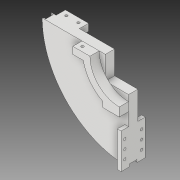
# Autodesk Inventor part: 2125B_Bearing Clamps Gear_V1
Saved by Autodesk Inventor 2020 (Build 240168000, 168)
## iProperties
Created: 2017-06-21
Part Number: 2125B_Bearing Clamps Gear_V1
Material: ABS Plastic
Document SubType Name: Modeling
Designer: MPI
Density: 1.06 g/cm^3
Appearance: Smooth - White
Mass: 4002.07 g
Surface Area: 3908.8 cm^2
Volume: 3775.53 cm^3
Author: MPI
Autodesk Inventor part; units mm, degrees
(part 1 of 3)
ref_plane "YZ Plane" through (0, 0, 0) normal (1, 0, 0) x (0, 1, 0)
ref_plane "XZ Plane" through (0, 0, 0) normal (0, 1, 0) x (-1, 0, 0)
ref_plane "XY Plane" through (0, 0, 0) normal (0, 0, 1) x (1, 0, 0)
sketch "Sketch1" plane through (0, 0, 0) normal (0, 0, 1) x (1, 0, 0)
  circle A0 centre (0, 0) radius 80.137
  line L0 (-127, -19.05) -> (-127, 19.05)
  line L1 (127, 19.05) -> (127, -19.05)
  line L2 (127, -19.05) -> (-127, 19.05) construction
  line L3 (-127, -19.05) -> (127, 19.05) construction
  line L4 (-127, 0) -> (88.9567, 0) construction
  line L5 (-127, 19.05) -> (-99.7981, 19.05)
  line L6 (99.7981, 19.05) -> (127, 19.05)
  arc A1 (-98.1276, -19.05) -> (98.1276, -19.05) centre (0, 0) ccw
  arc A2 (99.7981, 19.05) -> (-99.7981, 19.05) centre (0, 0) ccw
  line L7 (127, -19.05) -> (98.1276, -19.05)
  line L8 (-98.1276, -19.05) -> (-127, -19.05)
  dimension "d0" = 160.274
  dimension "d2" = 254
  dimension "d3" = 38.1
  dimension "d137" = 101.6
  dimension "d138" = 127
  dimension "d139" = 19.05
  dimension "d155" = 21.463
  constraints: 18 end point, 7 parallel, 4 point on circle, 3 centre point, 3 midpoint, 2 coincident, 2 horizontal, 2 perpendicular
  measures "d0" diameter of A0
  measures "d2" distance of L1.end L0.start
  measures "d3" distance of L0.start L0.end
  measures "d137" radius of A2
  measures "d138" distance from line of A0.centre L0
  measures "d139" distance from line of A0.centre L5
  measures "d155" radial gap between concentric circles of A2 A0
extrude "Extrusion1" add sketch "Sketch1" along normal blind 25.4
sketch "Sketch2" plane through (99.7981, 19.05, 0) normal (0, 1, 0) x (1, 0, 0)
  line L0 (27.2019, 0) -> (0, 0) projected
  line L1 (0, 0) -> (0, -25.4) projected
  line L2 (27.2019, -25.4) -> (0, -25.4) projected
  line L3 (27.2019, 0) -> (27.2019, -25.4) projected
  line L4 (27.2019, -12.7) -> (0, -12.7) construction
  line L5 (13.601, -25.4) -> (13.601, 0) construction
  circle A0 centre (13.601, -12.7) radius 3.3782
  point P0 (-99.7981, 0)
  dimension "d6" = 6.7564
  constraints: 5 midpoint, 4 end point, 1 centre point
  measures "d6" diameter of A0
extrude "Extrusion2" cut sketch "Sketch2" against normal blind 38.1 contours A0
mirror "Mirror1" about plane through (0, 0, 0) normal (1, 0, 0) of "Extrusion2"
sketch "Sketch4" plane through (0, 0, 0) normal (0, 0, -1) x (-1, 0, 0)
  arc A0 (99.7981, 19.05) -> (-99.7981, 19.05) centre (0, 0) ccw projected
  line L0 (-63.5, -63.5) -> (63.5, -63.5)
  line L1 (63.5, -63.5) -> (63.5, 63.5)
  line L2 (63.5, 63.5) -> (-63.5, 63.5)
  line L3 (-63.5, 63.5) -> (-63.5, -63.5)
  line L4 (-63.5, -63.5) -> (63.5, 63.5) construction
  line L5 (-89.8026, 89.8026) -> (89.8026, -89.8026) construction
  circle A1 centre (0, 0) radius 228.9048
  circle A2 centre (0, 0) radius 146.8598 construction
  line L6 (-9.525, 228.7065) -> (-6.111, 146.7326) construction
  line L7 (0, 146.8598) -> (0, 125.8958) construction
  arc A3 (0, 125.8958) -> (-4.7163, 125.8085) centre (-0.0298, 0.0716) ccw construction
  line L8 (-2.3813, 228.8924) -> (-2.3813, 146.8405)
  line L9 (-6.7286, 228.824) -> (-6.7278, 228.8059)
  arc A4 (-5.196, 124.7614) -> (-9.4765, 124.5104) centre (-0.0298, 0.0716) ccw
  arc A5 (-2.3813, 146.8405) -> (-4.0495, 146.8039) centre (0, 0) ccw
  line L10 (-7.1437, 228.7933) -> (-5.8965, 146.7413)
  dimension "d11" = 127
  dimension "d12" = 127
  dimension "d28" = 457.8096
  dimension "d30" = 82.045
  dimension "d33" = 9.525
  dimension "d34" = 20.964
  dimension "d35" = 81.974
  dimension "d36" = 2.3813
  dimension "d39" = 2.3813
  dimension "d40" = 82.052
  dimension "d41" = 82.052
  constraints: 22 end point, 15 point on circle, 5 centre point, 3 parallel, 2 coincident, 2 concentric, 2 line through centre, 2 midpoint, 1 horizontal, 1 perpendicular, 1 point on line, 1 vertical
  measures "d11" distance of L2.end L1.end
  measures "d12" distance of L1.end L0.end
  measures "d28" diameter of A1
  measures "d30" radial gap between concentric circles of A1 A2
  measures "d33" horizontal distance of L7.end L6.start
  measures "d34" distance of L7.start L7.end
  measures "d35" vertical distance of L6.start L6.end
  measures "d36" distance between parallel lines of L8 L7
  measures "d39" horizontal distance of L6.start L10.start
  measures "d40" distance of L8.start L8.end
  measures "d41" vertical distance of L10.start L10.end
extrude "Extrusion4" add sketch "Sketch4" along normal blind 25.4 separate body
sketch "Sketch8" plane through (0, 0, 0) normal (0, 0, 1) x (1, 0, 0)
  circle A0 centre (0, 0) radius 228.9048 projected
  arc A1 (9.5229, 228.7066) -> (0, 228.9048) centre (0, 0) ccw
  line L0 (4.7625, 228.8553) -> (4.7182, 226.7257) construction
  circle A2 centre (0, 0) radius 226.7801 construction
  line L1 (-6.0145, 226.7003) -> (3.1685, 226.758) construction
  line L2 (9.5229, 228.7066) -> (9.4345, 226.5838) construction
  line L3 (9.4345, 226.5838) -> (6.2678, 226.6935) construction
  line L4 (6.2678, 226.6935) -> (7.1073, 228.7944)
  line L5 (3.1685, 226.758) -> (2.4172, 228.892)
  arc A3 (99.7981, 19.05) -> (-99.7981, 19.05) centre (0, 0) ccw projected
  line L6 (7.1073, 228.7944) -> (0, 0) construction
  line L7 (0, 0) -> (2.4172, 228.892) construction
  line L8 (6.2678, 226.6935) -> (3.1685, 226.758)
  point P0 (12.7, 94.3995)
  point P1 (-12.7, 94.3995)
  dimension "d42" = 9.525
  dimension "d43" = 2.13
  dimension "d46" = 3.1686
  dimension "d52" = 20
  dimension "d53" = 20
  dimension "d55" = 3.1
  constraints: 18 end point, 13 point on circle, 2 centre point, 2 line through centre, 1 concentric, 1 midpoint, 1 vertical alignment, 1 other
  measures "d42" distance of A0.end L2.start
  measures "d43" distance of L0.end L0.start
  measures "d46" distance of L2.end L3.end
  measures "d52" angle of L5 L7
  measures "d53" angle of L6 L4
  measures "d55" distance of L1.end L3.end
extrude "Extrusion6" cut sketch "Sketch8" against normal blind 25.4 contours L4 L8 L5 A0 picked at (4.4724, 227.4406) bodies 2
pattern_circular "Circular Pattern1" count 152 over 360 about axis through (0, 0, 0) along (0, 0, -1) of "Extrusion6" bodies 2
sketch "Sketch9" plane through (0, 0, 25.4) normal (0, 0, 1) x (1, 0, 0)
  circle A0 centre (-78.9498, 78.9498) radius 4.7625 projected
  circle A1 centre (78.9498, 78.9498) radius 4.7625 projected
  line L0 (127, -19.05) -> (127, 19.05) projected
  line L1 (127, 19.05) -> (99.7981, 19.05) projected
  line L2 (94.3995, 12.7) -> (94.3995, 94.3995) projected
  line L3 (94.3995, 94.3995) -> (12.7, 94.3995) projected
  arc A2 (99.7981, 19.05) -> (-99.7981, 19.05) centre (0, 0) ccw projected
  line L4 (-12.7, 94.3995) -> (-94.3995, 94.3995) projected
  line L5 (-94.3995, 94.3995) -> (-94.3995, 12.7) projected
  line L6 (-99.7981, 19.05) -> (-127, 19.05) projected
  line L7 (-127, 19.05) -> (-127, -19.05) projected
  line L8 (-127, 0) -> (127, 0)
  constraints: 2 end point, 2 midpoint, 3 other
extrude "Extrusion7" cut sketch "Sketch9" against normal blind 25.4 contours L8 L7 L6 A2 L1 L0 bodies 1
sketch "Sketch11" plane through (0, 0, 0) normal (0, 0, 1) x (1, 0, 0)
  line L0 (-63.5, 63.5) -> (63.5, 63.5) projected
  line L1 (0, 63.5) -> (0, 139.7) construction
  line L2 (0, 63.5) -> (76.2, 63.5) construction
  line L3 (0, 139.7) -> (25.4, 139.7) construction
  line L4 (-25.4, 127) -> (25.4, 127) construction
  line L5 (25.4, 127) -> (25.4, 152.4)
  line L6 (25.4, 152.4) -> (-25.4, 152.4) construction
  line L7 (-25.4, 152.4) -> (-25.4, 127)
  line L8 (-25.4, 127) -> (25.4, 152.4) construction
  line L9 (25.4, 127) -> (-25.4, 152.4) construction
  line L10 (0, 139.7) -> (0, 133.35)
  line L11 (0, 133.35) -> (25.4, 127)
  line L12 (0, 133.35) -> (-25.4, 127)
  line L13 (0, 146.05) -> (25.4, 152.4)
  line L14 (0, 146.05) -> (-25.4, 152.4)
  line L15 (-25.4, 127) -> (-25.4, 107.95) construction
  line L16 (-25.4, 107.95) -> (25.4, 107.95) construction
  circle A0 centre (-25.4, 107.95) radius 4.4323
  circle A1 centre (25.4, 107.95) radius 4.4323
  line L17 (-25.4, 139.7) -> (25.4, 139.7) construction
  circle A2 centre (-25.4, 171.45) radius 4.4323
  circle A3 centre (25.4, 171.45) radius 4.4323
  dimension "d65" = 76.2
  dimension "d66" = 90
  dimension "d67" = 25.4
  dimension "d68" = 25.4
  dimension "d69" = 6.35
  dimension "d127" = 19.05
  dimension "d128" = 50.8
  dimension "d129" = 90
  dimension "d130" = 8.8646
  dimension "d131" = 8.8646
  dimension "d132" = 25.4
  constraints: 34 end point, 4 centre point, 4 midpoint, 4 perpendicular, 3 parallel, 3 symmetric about line, 2 coincident, 2 vertical, 1 collinear, 1 horizontal, 1 point on line, 2 other
  measures "d65" distance of L1.start L1.end
  measures "d66" angle of L2 L1
  measures "d67" distance of L1.end L3.end
  measures "d68" distance of L5.end L4.end
  measures "d69" distance of L1.end L10.end
  measures "d127" distance of L4.start L15.end
  measures "d128" distance of L15.end L16.end
  measures "d129" angle of L16 L15
  measures "d130" diameter of A0
  measures "d131" diameter of A1
  measures "d132" distance from line of L16.end L1
extrude "Extrusion9" cut sketch "Sketch11" against normal blind 21.59 contours L11 L12 L7 L14 L13 L5 | A2 | A3 bodies 2
sketch "Sketch17" plane through (0, 0, 0) normal (0, 0, 1) x (1, 0, 0)
  line L0 (-15.5678, 226.2451) -> (-16.4928, 228.3099) projected
  arc A0 (-16.4928, 228.3099) -> (-21.2475, 227.9165) centre (0, 0) ccw projected
  line L1 (-21.2475, 227.9165) -> (-21.8206, 225.7279) projected
  line L2 (-21.8206, 225.7279) -> (-24.9041, 225.4085) projected
  line L3 (-24.9041, 225.4085) -> (-25.9136, 227.4333) projected
  arc A1 (-25.9136, 227.4333) -> (-30.648, 226.8438) centre (0, 0) ccw projected
  line L4 (-30.648, 226.8438) -> (-31.1302, 224.6333) projected
  line L5 (-31.1302, 224.6333) -> (-34.1978, 224.1868) projected
  line L6 (-34.1978, 224.1868) -> (-35.2902, 226.1681) projected
  arc A2 (-35.2902, 226.1681) -> (-39.9961, 225.3835) centre (0, 0) ccw projected
  line L7 (-39.9961, 225.3835) -> (-40.3865, 223.155) projected
  line L8 (-40.3865, 223.155) -> (-43.4331, 222.5821) projected
  line L9 (-43.4331, 222.5821) -> (-44.6064, 224.5165) projected
  arc A3 (-44.6064, 224.5165) -> (-49.2759, 223.5381) centre (0, 0) ccw projected
  line L10 (-49.2759, 223.5381) -> (-49.5739, 221.2954) projected
  line L11 (-49.5739, 221.2954) -> (-52.5942, 220.5971) projected
  line L12 (-52.5942, 220.5971) -> (-53.8464, 222.4814) projected
  arc A4 (-53.8464, 222.4814) -> (-58.4715, 221.3108) centre (0, 0) ccw projected
  line L13 (-58.4715, 221.3108) -> (-58.6766, 219.0577) projected
  line L14 (-58.6766, 219.0577) -> (-61.6655, 218.2352) projected
  line L15 (-61.6655, 218.2352) -> (-62.9945, 220.0661) projected
  arc A5 (-62.9945, 220.0661) -> (-67.5672, 218.7055) centre (0, 0) ccw projected
  line L16 (-67.5672, 218.7055) -> (-67.679, 216.4458) projected
  line L17 (-67.679, 216.4458) -> (-70.6313, 215.5004) projected
  line L18 (-70.6313, 215.5004) -> (-72.0349, 217.2749) projected
  arc A6 (-72.0349, 217.2749) -> (-76.5475, 215.7264) centre (0, 0) ccw projected
  line L19 (-76.5475, 215.7264) -> (-76.5658, 213.464) projected
  line L20 (-76.5658, 213.464) -> (-79.4766, 212.3975) projected
  line L21 (-79.4766, 212.3975) -> (-80.9522, 214.1125) projected
  arc A7 (-80.9522, 214.1125) -> (-85.397, 212.3788) centre (0, 0) ccw projected
  line L22 (-85.397, 212.3788) -> (-85.3218, 210.1176) projected
  line L23 (-85.3218, 210.1176) -> (-88.186, 208.9317) projected
  line L24 (-88.186, 208.9317) -> (-89.7313, 210.5842) projected
  arc A8 (-89.7313, 210.5842) -> (-94.1006, 208.6684) centre (0, 0) ccw projected
  line L25 (-94.1006, 208.6684) -> (-93.932, 206.4122) projected
  line L26 (-93.932, 206.4122) -> (-96.7448, 205.1089) projected
  line L27 (-96.7448, 205.1089) -> (-98.357, 206.6962) projected
  arc A9 (-98.357, 206.6962) -> (-102.6434, 204.6014) centre (0, 0) ccw projected
  line L28 (-102.6434, 204.6014) -> (-102.3818, 202.3541) projected
  line L29 (-102.3818, 202.3541) -> (-105.1382, 200.9357) projected
  line L30 (-105.1382, 200.9357) -> (-106.8147, 202.455) projected
  arc A10 (-106.8147, 202.455) -> (-111.0109, 200.1849) centre (0, 0) ccw projected
  line L31 (-111.0109, 200.1849) -> (-110.6566, 197.9503) projected
  line L32 (-110.6566, 197.9503) -> (-113.3521, 196.4192) projected
  line L33 (-113.3521, 196.4192) -> (-115.0899, 197.8679) projected
  arc A11 (-115.0899, 197.8679) -> (-119.1887, 195.4264) centre (0, 0) ccw projected
  line L34 (-119.1887, 195.4264) -> (-118.7423, 193.2084) projected
  line L35 (-118.7423, 193.2084) -> (-121.3723, 191.5672) projected
  line L36 (-121.3723, 191.5672) -> (-123.1685, 192.9428) projected
  arc A12 (-123.1685, 192.9428) -> (-127.1629, 190.3339) centre (0, 0) ccw projected
  line L37 (-127.1629, 190.3339) -> (-126.6252, 188.1363) projected
  line L38 (-126.6252, 188.1363) -> (-129.1851, 186.3878) projected
  line L39 (-129.1851, 186.3878) -> (-131.0366, 187.6881) projected
  arc A13 (-131.0366, 187.6881) -> (-134.9198, 184.9163) centre (0, 0) ccw projected
  line L40 (-134.9198, 184.9163) -> (-134.2918, 182.7428) projected
  line L41 (-134.2918, 182.7428) -> (-136.7772, 180.89) projected
  line L42 (-136.7772, 180.89) -> (-138.6809, 182.1127) projected
  arc A14 (-138.6809, 182.1127) -> (-142.4462, 179.1828) centre (0, 0) ccw projected
  line L43 (-142.4462, 179.1828) -> (-141.7289, 177.0371) projected
  line L44 (-141.7289, 177.0371) -> (-144.1357, 175.0832) projected
  line L45 (-144.1357, 175.0832) -> (-146.0882, 176.2261) projected
  arc A15 (-146.0882, 176.2261) -> (-149.7292, 173.1432) centre (0, 0) ccw projected
  line L46 (-149.7292, 173.1432) -> (-148.9239, 171.0289) projected
  line L47 (-148.9239, 171.0289) -> (-151.2478, 168.9772) projected
  line L48 (-151.2478, 168.9772) -> (-153.246, 170.0385) projected
  arc A16 (-153.246, 170.0385) -> (-156.7565, 166.8077) centre (0, 0) ccw projected
  line L49 (-156.7565, 166.8077) -> (-155.8644, 164.7285) projected
  line L50 (-155.8644, 164.7285) -> (-158.1016, 162.5826) projected
  line L51 (-158.1016, 162.5826) -> (-160.1419, 163.5603) projected
  arc A17 (-160.1419, 163.5603) -> (-163.5159, 160.1873) centre (0, 0) ccw projected
  line L52 (-163.5159, 160.1873) -> (-162.5387, 158.1467) projected
  line L53 (-162.5387, 158.1467) -> (-164.6853, 155.9101) projected
  line L54 (-164.6853, 155.9101) -> (-166.7642, 156.8028) projected
  arc A18 (-166.7642, 156.8028) -> (-169.9959, 153.2931) centre (0, 0) ccw projected
  line L55 (-169.9959, 153.2931) -> (-168.9353, 151.2947) projected
  line L56 (-168.9353, 151.2947) -> (-170.9876, 148.9713) projected
  line L57 (-170.9876, 148.9713) -> (-173.1016, 149.7773) projected
  arc A19 (-173.1016, 149.7773) -> (-176.1856, 146.1371) centre (0, 0) ccw projected
  line L58 (-176.1856, 146.1371) -> (-175.0432, 144.1842) projected
  line L59 (-175.0432, 144.1842) -> (-176.9977, 141.778) projected
  line L60 (-176.9977, 141.778) -> (-179.1433, 142.4959) projected
  arc A20 (-179.1433, 142.4959) -> (-182.0742, 138.7314) centre (0, 0) ccw projected
  line L61 (-182.0742, 138.7314) -> (-180.8521, 136.8274) projected
  line L62 (-180.8521, 136.8274) -> (-182.7055, 134.3425) projected
  line L63 (-182.7055, 134.3425) -> (-184.8789, 134.9711) projected
  arc A21 (-184.8789, 134.9711) -> (-187.6517, 131.0887) centre (0, 0) ccw projected
  line L64 (-187.6517, 131.0887) -> (-186.352, 129.2368) projected
  line L65 (-186.352, 129.2368) -> (-188.1011, 126.6774) projected
  line L66 (-188.1011, 126.6774) -> (-190.2987, 127.2157) projected
  arc A22 (-190.2987, 127.2157) -> (-192.9086, 123.222) centre (0, 0) ccw projected
  line L67 (-192.9086, 123.222) -> (-191.5335, 121.4254) projected
  line L68 (-191.5335, 121.4254) -> (-193.1754, 118.7959) projected
  line L69 (-193.1754, 118.7959) -> (-195.3933, 119.2429) projected
  arc A23 (-195.3933, 119.2429) -> (-197.836, 115.1448) centre (0, 0) ccw projected
  line L70 (-197.836, 115.1448) -> (-196.3878, 113.4066) projected
  line L71 (-196.3878, 113.4066) -> (-197.9196, 110.7115) projected
  line L72 (-197.9196, 110.7115) -> (-200.1541, 111.0664) projected
  arc A24 (-200.1541, 111.0664) -> (-202.4254, 106.8709) centre (0, 0) ccw projected
  line L73 (-202.4254, 106.8709) -> (-200.9065, 105.194) projected
  line L74 (-200.9065, 105.194) -> (-202.3257, 102.4379) projected
  line L75 (-202.3257, 102.4379) -> (-204.5729, 102.7002) projected
  arc A25 (-204.5729, 102.7002) -> (-206.6689, 98.4143) centre (0, 0) ccw projected
  line L76 (-206.6689, 98.4143) -> (-205.0821, 96.8017) projected
  line L77 (-205.0821, 96.8017) -> (-206.3861, 93.9893) projected
  line L78 (-206.3861, 93.9893) -> (-208.6422, 94.1585) projected
  arc A26 (-208.6422, 94.1585) -> (-210.5593, 89.7897) centre (0, 0) ccw projected
  line L79 (-210.5593, 89.7897) -> (-208.9072, 88.244) projected
  line L80 (-208.9072, 88.244) -> (-210.0939, 85.3801) projected
  line L81 (-210.0939, 85.3801) -> (-212.3551, 85.4559) projected
  arc A27 (-212.3551, 85.4559) -> (-214.09, 81.0116) centre (0, 0) ccw projected
  line L82 (-214.09, 81.0116) -> (-212.3754, 79.5355) projected
  line L83 (-212.3754, 79.5355) -> (-213.4428, 76.625) projected
  line L84 (-213.4428, 76.625) -> (-215.7052, 76.6074) projected
  arc A28 (-215.7052, 76.6074) -> (-217.2549, 72.0952) centre (0, 0) ccw projected
  line L85 (-217.2549, 72.0952) -> (-215.4808, 70.6911) projected
  line L86 (-215.4808, 70.6911) -> (-216.427, 67.7391) projected
  line L87 (-216.427, 67.7391) -> (-218.6867, 67.6279) projected
  arc A29 (-218.6867, 67.6279) -> (-220.0486, 63.0555) centre (0, 0) ccw projected
  line L88 (-220.0486, 63.0555) -> (-218.218, 61.726) projected
  line L89 (-218.218, 61.726) -> (-219.0414, 58.7374) projected
  line L90 (-219.0414, 58.7374) -> (-221.2946, 58.5329) projected
  arc A30 (-221.2946, 58.5329) -> (-222.4664, 53.9082) centre (0, 0) ccw projected
  line L91 (-222.4664, 53.9082) -> (-220.5825, 52.6554) projected
  line L92 (-220.5825, 52.6554) -> (-221.2816, 49.6353) projected
  line L93 (-221.2816, 49.6353) -> (-223.5244, 49.3379) projected
  arc A31 (-223.5244, 49.3379) -> (-224.5042, 44.6687) centre (0, 0) ccw projected
  line L94 (-224.5042, 44.6687) -> (-222.57, 43.4949) projected
  line L95 (-222.57, 43.4949) -> (-223.1438, 40.4484) projected
  line L96 (-223.1438, 40.4484) -> (-225.3724, 40.0586) projected
  arc A32 (-225.3724, 40.0586) -> (-226.1583, 35.3529) centre (0, 0) ccw projected
  line L97 (-226.1583, 35.3529) -> (-224.1773, 34.26) projected
  line L98 (-224.1773, 34.26) -> (-224.6247, 31.1925) projected
  line L99 (-224.6247, 31.1925) -> (-226.8353, 30.7109) projected
  arc A33 (-226.8353, 30.7109) -> (-227.4261, 25.9767) centre (0, 0) ccw projected
  line L100 (-227.4261, 25.9767) -> (-225.4016, 24.9666) projected
  line L101 (-225.4016, 24.9666) -> (-225.7218, 21.8832) projected
  line L102 (-225.7218, 21.8832) -> (-227.9106, 21.3107) projected
  arc A34 (-227.9106, 21.3107) -> (-228.3053, 16.5561) centre (0, 0) ccw projected
  line L103 (-228.3053, 16.5561) -> (-226.2408, 15.6306) projected
  line L104 (-226.2408, 15.6306) -> (-226.4333, 12.5366) projected
  line L105 (-226.4333, 12.5366) -> (-228.5966, 11.8741) projected
  arc A35 (-228.5966, 11.8741) -> (-228.7944, 7.1073) centre (0, 0) ccw projected
  line L106 (-228.7944, 7.1073) -> (-226.6935, 6.2678) projected
  line L107 (-226.6935, 6.2678) -> (-226.758, 3.1685) projected
  line L108 (-226.758, 3.1685) -> (-228.892, 2.4172) projected
  arc A36 (-228.892, 2.4172) -> (-228.8927, -2.3537) centre (0, 0) ccw projected
  line L109 (-228.8927, -2.3537) -> (-226.7588, -3.1056) projected
  line L110 (-226.7588, -3.1056) -> (-226.6952, -6.205) projected
  line L111 (-226.6952, -6.205) -> (-228.7964, -7.0438) projected
  arc A37 (-228.7964, -7.0438) -> (-228.5999, -11.8107) centre (0, 0) ccw projected
  line L112 (-228.5999, -11.8107) -> (-226.4368, -12.4738) projected
  line L113 (-226.4368, -12.4738) -> (-226.2451, -15.5678) projected
  line L114 (-226.2451, -15.5678) -> (-228.3099, -16.4928) projected
  arc A38 (-228.3099, -16.4928) -> (-227.9165, -21.2475) centre (0, 0) ccw projected
  line L115 (-227.9165, -21.2475) -> (-225.7279, -21.8206) projected
  line L116 (-225.7279, -21.8206) -> (-225.4085, -24.9041) projected
  line L117 (-225.4085, -24.9041) -> (-227.4333, -25.9136) projected
  arc A39 (-227.4333, -25.9136) -> (-226.8438, -30.648) centre (0, 0) ccw projected
  line L118 (-226.8438, -30.648) -> (-224.6333, -31.1302) projected
  line L119 (-224.6333, -31.1302) -> (-224.1868, -34.1978) projected
  line L120 (-224.1868, -34.1978) -> (-226.1681, -35.2902) projected
  arc A40 (-226.1681, -35.2902) -> (-225.3835, -39.9961) centre (0, 0) ccw projected
  line L121 (-225.3835, -39.9961) -> (-223.155, -40.3865) projected
  line L122 (-223.155, -40.3865) -> (-222.5821, -43.4331) projected
  line L123 (-222.5821, -43.4331) -> (-224.5165, -44.6064) projected
  arc A41 (-224.5165, -44.6064) -> (-223.5381, -49.2759) centre (0, 0) ccw projected
  line L124 (-223.5381, -49.2759) -> (-221.2954, -49.5739) projected
  line L125 (-221.2954, -49.5739) -> (-220.5971, -52.5942) projected
  line L126 (-220.5971, -52.5942) -> (-222.4814, -53.8464) projected
  arc A42 (-222.4814, -53.8464) -> (-221.3108, -58.4715) centre (0, 0) ccw projected
  line L127 (-221.3108, -58.4715) -> (-219.0577, -58.6766) projected
  line L128 (-219.0577, -58.6766) -> (-218.2352, -61.6655) projected
  line L129 (-218.2352, -61.6655) -> (-220.0661, -62.9945) projected
  arc A43 (-220.0661, -62.9945) -> (-218.7055, -67.5672) centre (0, 0) ccw projected
  line L130 (-218.7055, -67.5672) -> (-216.4458, -67.679) projected
  line L131 (-216.4458, -67.679) -> (-215.5004, -70.6313) projected
  line L132 (-215.5004, -70.6313) -> (-217.2749, -72.0349) projected
  arc A44 (-217.2749, -72.0349) -> (-215.7264, -76.5475) centre (0, 0) ccw projected
  line L133 (-215.7264, -76.5475) -> (-213.464, -76.5658) projected
  line L134 (-213.464, -76.5658) -> (-212.3975, -79.4766) projected
  line L135 (-212.3975, -79.4766) -> (-214.1125, -80.9522) projected
  arc A45 (-214.1125, -80.9522) -> (-212.3788, -85.397) centre (0, 0) ccw projected
  line L136 (-212.3788, -85.397) -> (-210.1176, -85.3218) projected
  line L137 (-210.1176, -85.3218) -> (-208.9317, -88.186) projected
  line L138 (-208.9317, -88.186) -> (-210.5842, -89.7313) projected
  arc A46 (-210.5842, -89.7313) -> (-208.6684, -94.1006) centre (0, 0) ccw projected
  line L139 (-208.6684, -94.1006) -> (-206.4122, -93.932) projected
  line L140 (-206.4122, -93.932) -> (-205.1089, -96.7448) projected
  line L141 (-205.1089, -96.7448) -> (-206.6962, -98.357) projected
  arc A47 (-206.6962, -98.357) -> (-204.6014, -102.6434) centre (0, 0) ccw projected
  line L142 (-204.6014, -102.6434) -> (-202.3541, -102.3818) projected
  line L143 (-202.3541, -102.3818) -> (-200.9357, -105.1382) projected
  line L144 (-200.9357, -105.1382) -> (-202.455, -106.8147) projected
  arc A48 (-202.455, -106.8147) -> (-200.1849, -111.0109) centre (0, 0) ccw projected
  line L145 (-200.1849, -111.0109) -> (-197.9503, -110.6566) projected
  line L146 (-197.9503, -110.6566) -> (-196.4192, -113.3521) projected
  line L147 (-196.4192, -113.3521) -> (-197.8679, -115.0899) projected
  arc A49 (-197.8679, -115.0899) -> (-195.4264, -119.1887) centre (0, 0) ccw projected
  line L148 (-195.4264, -119.1887) -> (-193.2084, -118.7423) projected
  line L149 (-193.2084, -118.7423) -> (-191.5672, -121.3723) projected
  line L150 (-191.5672, -121.3723) -> (-192.9428, -123.1685) projected
  arc A50 (-192.9428, -123.1685) -> (-190.3339, -127.1629) centre (0, 0) ccw projected
  line L151 (-190.3339, -127.1629) -> (-188.1363, -126.6252) projected
  line L152 (-188.1363, -126.6252) -> (-186.3878, -129.1851) projected
  line L153 (-186.3878, -129.1851) -> (-187.6881, -131.0366) projected
  arc A51 (-187.6881, -131.0366) -> (-184.9163, -134.9198) centre (0, 0) ccw projected
  line L154 (-184.9163, -134.9198) -> (-182.7428, -134.2918) projected
  line L155 (-182.7428, -134.2918) -> (-180.89, -136.7772) projected
  line L156 (-180.89, -136.7772) -> (-182.1127, -138.6809) projected
  arc A52 (-182.1127, -138.6809) -> (-179.1828, -142.4462) centre (0, 0) ccw projected
  line L157 (-179.1828, -142.4462) -> (-177.0371, -141.7289) projected
  line L158 (-177.0371, -141.7289) -> (-175.0832, -144.1357) projected
  line L159 (-175.0832, -144.1357) -> (-176.2261, -146.0882) projected
  arc A53 (-176.2261, -146.0882) -> (-173.1432, -149.7292) centre (0, 0) ccw projected
  line L160 (-173.1432, -149.7292) -> (-171.0289, -148.9239) projected
  line L161 (-171.0289, -148.9239) -> (-168.9772, -151.2478) projected
  line L162 (-168.9772, -151.2478) -> (-170.0385, -153.246) projected
  arc A54 (-170.0385, -153.246) -> (-166.8077, -156.7565) centre (0, 0) ccw projected
  line L163 (-166.8077, -156.7565) -> (-164.7285, -155.8644) projected
  line L164 (-164.7285, -155.8644) -> (-162.5826, -158.1016) projected
  line L165 (-162.5826, -158.1016) -> (-163.5603, -160.1419) projected
  arc A55 (-163.5603, -160.1419) -> (-160.1873, -163.5159) centre (0, 0) ccw projected
  line L166 (-160.1873, -163.5159) -> (-158.1467, -162.5387) projected
  line L167 (-158.1467, -162.5387) -> (-155.9101, -164.6853) projected
  line L168 (-155.9101, -164.6853) -> (-156.8028, -166.7642) projected
  arc A56 (-156.8028, -166.7642) -> (-153.2931, -169.9959) centre (0, 0) ccw projected
  line L169 (-153.2931, -169.9959) -> (-151.2947, -168.9353) projected
  line L170 (-151.2947, -168.9353) -> (-148.9713, -170.9876) projected
  line L171 (-148.9713, -170.9876) -> (-149.7773, -173.1016) projected
  arc A57 (-149.7773, -173.1016) -> (-146.1371, -176.1856) centre (0, 0) ccw projected
  line L172 (-146.1371, -176.1856) -> (-144.1842, -175.0432) projected
  line L173 (-144.1842, -175.0432) -> (-141.778, -176.9977) projected
  line L174 (-141.778, -176.9977) -> (-142.4959, -179.1433) projected
  arc A58 (-142.4959, -179.1433) -> (-138.7314, -182.0742) centre (0, 0) ccw projected
  line L175 (-138.7314, -182.0742) -> (-136.8274, -180.8521) projected
  line L176 (-136.8274, -180.8521) -> (-134.3425, -182.7055) projected
  line L177 (-134.3425, -182.7055) -> (-134.9711, -184.8789) projected
  arc A59 (-134.9711, -184.8789) -> (-131.0887, -187.6517) centre (0, 0) ccw projected
  line L178 (-131.0887, -187.6517) -> (-129.2368, -186.352) projected
  line L179 (-129.2368, -186.352) -> (-126.6774, -188.1011) projected
  line L180 (-126.6774, -188.1011) -> (-127.2157, -190.2987) projected
  arc A60 (-127.2157, -190.2987) -> (-123.222, -192.9086) centre (0, 0) ccw projected
  line L181 (-123.222, -192.9086) -> (-121.4254, -191.5335) projected
  line L182 (-121.4254, -191.5335) -> (-118.7959, -193.1754) projected
  line L183 (-118.7959, -193.1754) -> (-119.2429, -195.3933) projected
  arc A61 (-119.2429, -195.3933) -> (-115.1448, -197.836) centre (0, 0) ccw projected
  line L184 (-115.1448, -197.836) -> (-113.4066, -196.3878) projected
  line L185 (-113.4066, -196.3878) -> (-110.7115, -197.9196) projected
  line L186 (-110.7115, -197.9196) -> (-111.0664, -200.1541) projected
  arc A62 (-111.0664, -200.1541) -> (-106.8709, -202.4254) centre (0, 0) ccw projected
  line L187 (-106.8709, -202.4254) -> (-105.194, -200.9065) projected
  line L188 (-105.194, -200.9065) -> (-102.4379, -202.3257) projected
  line L189 (-102.4379, -202.3257) -> (-102.7002, -204.5729) projected
  arc A63 (-102.7002, -204.5729) -> (-98.4143, -206.6689) centre (0, 0) ccw projected
  line L190 (-98.4143, -206.6689) -> (-96.8017, -205.0821) projected
  line L191 (-96.8017, -205.0821) -> (-93.9893, -206.3861) projected
  line L192 (-93.9893, -206.3861) -> (-94.1585, -208.6422) projected
  arc A64 (-94.1585, -208.6422) -> (-89.7897, -210.5593) centre (0, 0) ccw projected
  line L193 (-89.7897, -210.5593) -> (-88.244, -208.9072) projected
  line L194 (-88.244, -208.9072) -> (-85.3801, -210.0939) projected
  line L195 (-85.3801, -210.0939) -> (-85.4559, -212.3551) projected
  arc A65 (-85.4559, -212.3551) -> (-81.0116, -214.09) centre (0, 0) ccw projected
  line L196 (-81.0116, -214.09) -> (-79.5355, -212.3754) projected
  line L197 (-79.5355, -212.3754) -> (-76.625, -213.4428) projected
  line L198 (-76.625, -213.4428) -> (-76.6074, -215.7052) projected
  arc A66 (-76.6074, -215.7052) -> (-72.0952, -217.2549) centre (0, 0) ccw projected
  line L199 (-72.0952, -217.2549) -> (-70.6911, -215.4808) projected
  line L200 (-70.6911, -215.4808) -> (-67.7391, -216.427) projected
  line L201 (-67.7391, -216.427) -> (-67.6279, -218.6867) projected
  arc A67 (-67.6279, -218.6867) -> (-63.0555, -220.0486) centre (0, 0) ccw projected
  line L202 (-63.0555, -220.0486) -> (-61.726, -218.218) projected
  line L203 (-61.726, -218.218) -> (-58.7374, -219.0414) projected
  line L204 (-58.7374, -219.0414) -> (-58.5329, -221.2946) projected
  arc A68 (-58.5329, -221.2946) -> (-53.9082, -222.4664) centre (0, 0) ccw projected
  line L205 (-53.9082, -222.4664) -> (-52.6554, -220.5825) projected
  line L206 (-52.6554, -220.5825) -> (-49.6353, -221.2816) projected
  line L207 (-49.6353, -221.2816) -> (-49.3379, -223.5244) projected
  arc A69 (-49.3379, -223.5244) -> (-44.6687, -224.5042) centre (0, 0) ccw projected
  line L208 (-44.6687, -224.5042) -> (-43.4949, -222.57) projected
  line L209 (-43.4949, -222.57) -> (-40.4484, -223.1438) projected
  line L210 (-40.4484, -223.1438) -> (-40.0586, -225.3724) projected
  arc A70 (-40.0586, -225.3724) -> (-35.3529, -226.1583) centre (0, 0) ccw projected
  line L211 (-35.3529, -226.1583) -> (-34.26, -224.1773) projected
  line L212 (-34.26, -224.1773) -> (-31.1925, -224.6247) projected
  line L213 (-31.1925, -224.6247) -> (-30.7109, -226.8353) projected
  arc A71 (-30.7109, -226.8353) -> (-25.9767, -227.4261) centre (0, 0) ccw projected
  line L214 (-25.9767, -227.4261) -> (-24.9666, -225.4016) projected
  line L215 (-24.9666, -225.4016) -> (-21.8832, -225.7218) projected
  line L216 (-21.8832, -225.7218) -> (-21.3107, -227.9106) projected
  arc A72 (-21.3107, -227.9106) -> (-16.5561, -228.3053) centre (0, 0) ccw projected
  line L217 (-16.5561, -228.3053) -> (-15.6306, -226.2408) projected
  line L218 (-15.6306, -226.2408) -> (-12.5366, -226.4333) projected
  line L219 (-12.5366, -226.4333) -> (-11.8741, -228.5966) projected
  arc A73 (-11.8741, -228.5966) -> (-7.1073, -228.7944) centre (0, 0) ccw projected
  line L220 (-7.1073, -228.7944) -> (-6.2678, -226.6935) projected
  line L221 (-6.2678, -226.6935) -> (-3.1685, -226.758) projected
  line L222 (-3.1685, -226.758) -> (-2.4172, -228.892) projected
  arc A74 (-2.4172, -228.892) -> (2.3537, -228.8927) centre (0, 0) ccw projected
  line L223 (2.3537, -228.8927) -> (3.1056, -226.7588) projected
  line L224 (3.1056, -226.7588) -> (6.205, -226.6952) projected
  line L225 (6.205, -226.6952) -> (7.0438, -228.7964) projected
  arc A75 (7.0438, -228.7964) -> (11.8107, -228.5999) centre (0, 0) ccw projected
  line L226 (11.8107, -228.5999) -> (12.4738, -226.4368) projected
  line L227 (12.4738, -226.4368) -> (15.5678, -226.2451) projected
  line L228 (15.5678, -226.2451) -> (16.4928, -228.3099) projected
  arc A76 (16.4928, -228.3099) -> (21.2475, -227.9165) centre (0, 0) ccw projected
  line L229 (21.2475, -227.9165) -> (21.8206, -225.7279) projected
  line L230 (21.8206, -225.7279) -> (24.9041, -225.4085) projected
  line L231 (24.9041, -225.4085) -> (25.9136, -227.4333) projected
  arc A77 (25.9136, -227.4333) -> (30.648, -226.8438) centre (0, 0) ccw projected
  line L232 (30.648, -226.8438) -> (31.1302, -224.6333) projected
  line L233 (31.1302, -224.6333) -> (34.1978, -224.1868) projected
  line L234 (34.1978, -224.1868) -> (35.2902, -226.1681) projected
  arc A78 (35.2902, -226.1681) -> (39.9961, -225.3835) centre (0, 0) ccw projected
  line L235 (39.9961, -225.3835) -> (40.3865, -223.155) projected
  line L236 (40.3865, -223.155) -> (43.4331, -222.5821) projected
  line L237 (43.4331, -222.5821) -> (44.6064, -224.5165) projected
  arc A79 (44.6064, -224.5165) -> (49.2759, -223.5381) centre (0, 0) ccw projected
  line L238 (49.2759, -223.5381) -> (49.5739, -221.2954) projected
  line L239 (49.5739, -221.2954) -> (52.5942, -220.5971) projected
  line L240 (52.5942, -220.5971) -> (53.8464, -222.4814) projected
  arc A80 (53.8464, -222.4814) -> (58.4715, -221.3108) centre (0, 0) ccw projected
  line L241 (58.4715, -221.3108) -> (58.6766, -219.0577) projected
  line L242 (58.6766, -219.0577) -> (61.6655, -218.2352) projected
  line L243 (61.6655, -218.2352) -> (62.9945, -220.0661) projected
  arc A81 (62.9945, -220.0661) -> (67.5672, -218.7055) centre (0, 0) ccw projected
  line L244 (67.5672, -218.7055) -> (67.679, -216.4458) projected
  line L245 (67.679, -216.4458) -> (70.6313, -215.5004) projected
  line L246 (70.6313, -215.5004) -> (72.0349, -217.2749) projected
  arc A82 (72.0349, -217.2749) -> (76.5475, -215.7264) centre (0, 0) ccw projected
  line L247 (76.5475, -215.7264) -> (76.5658, -213.464) projected
  line L248 (76.5658, -213.464) -> (79.4766, -212.3975) projected
  line L249 (79.4766, -212.3975) -> (80.9522, -214.1125) projected
  arc A83 (80.9522, -214.1125) -> (85.397, -212.3788) centre (0, 0) ccw projected
  line L250 (85.397, -212.3788) -> (85.3218, -210.1176) projected
  line L251 (85.3218, -210.1176) -> (88.186, -208.9317) projected
  line L252 (88.186, -208.9317) -> (89.7313, -210.5842) projected
  arc A84 (89.7313, -210.5842) -> (94.1006, -208.6684) centre (0, 0) ccw projected
  line L253 (94.1006, -208.6684) -> (93.932, -206.4122) projected
  line L254 (93.932, -206.4122) -> (96.7448, -205.1089) projected
  line L255 (96.7448, -205.1089) -> (98.357, -206.6962) projected
  arc A85 (98.357, -206.6962) -> (102.6434, -204.6014) centre (0, 0) ccw projected
  line L256 (102.6434, -204.6014) -> (102.3818, -202.3541) projected
  line L257 (102.3818, -202.3541) -> (105.1382, -200.9357) projected
  line L258 (105.1382, -200.9357) -> (106.8147, -202.455) projected
  arc A86 (106.8147, -202.455) -> (111.0109, -200.1849) centre (0, 0) ccw projected
  line L259 (111.0109, -200.1849) -> (110.6566, -197.9503) projected
  line L260 (110.6566, -197.9503) -> (113.3521, -196.4192) projected
  line L261 (113.3521, -196.4192) -> (115.0899, -197.8679) projected
  arc A87 (115.0899, -197.8679) -> (119.1887, -195.4264) centre (0, 0) ccw projected
  line L262 (119.1887, -195.4264) -> (118.7423, -193.2084) projected
  line L263 (118.7423, -193.2084) -> (121.3723, -191.5672) projected
  line L264 (121.3723, -191.5672) -> (123.1685, -192.9428) projected
  arc A88 (123.1685, -192.9428) -> (127.1629, -190.3339) centre (0, 0) ccw projected
  line L265 (127.1629, -190.3339) -> (126.6252, -188.1363) projected
  line L266 (126.6252, -188.1363) -> (129.1851, -186.3878) projected
  line L267 (129.1851, -186.3878) -> (131.0366, -187.6881) projected
  arc A89 (131.0366, -187.6881) -> (134.9198, -184.9163) centre (0, 0) ccw projected
  line L268 (134.9198, -184.9163) -> (134.2918, -182.7428) projected
  line L269 (134.2918, -182.7428) -> (136.7772, -180.89) projected
  line L270 (136.7772, -180.89) -> (138.6809, -182.1127) projected
  arc A90 (138.6809, -182.1127) -> (142.4462, -179.1828) centre (0, 0) ccw projected
  line L271 (142.4462, -179.1828) -> (141.7289, -177.0371) projected
  line L272 (141.7289, -177.0371) -> (144.1357, -175.0832) projected
  line L273 (144.1357, -175.0832) -> (146.0882, -176.2261) projected
  arc A91 (146.0882, -176.2261) -> (149.7292, -173.1432) centre (0, 0) ccw projected
  line L274 (149.7292, -173.1432) -> (148.9239, -171.0289) projected
  line L275 (148.9239, -171.0289) -> (151.2478, -168.9772) projected
  line L276 (151.2478, -168.9772) -> (153.246, -170.0385) projected
  arc A92 (153.246, -170.0385) -> (156.7565, -166.8077) centre (0, 0) ccw projected
  line L277 (156.7565, -166.8077) -> (155.8644, -164.7285) projected
  line L278 (155.8644, -164.7285) -> (158.1016, -162.5826) projected
  line L279 (158.1016, -162.5826) -> (160.1419, -163.5603) projected
  arc A93 (160.1419, -163.5603) -> (163.5159, -160.1873) centre (0, 0) ccw projected
  line L280 (163.5159, -160.1873) -> (162.5387, -158.1467) projected
  line L281 (162.5387, -158.1467) -> (164.6853, -155.9101) projected
  line L282 (164.6853, -155.9101) -> (166.7642, -156.8028) projected
  arc A94 (166.7642, -156.8028) -> (169.9959, -153.2931) centre (0, 0) ccw projected
  line L283 (169.9959, -153.2931) -> (168.9353, -151.2947) projected
  line L284 (168.9353, -151.2947) -> (170.9876, -148.9713) projected
  line L285 (170.9876, -148.9713) -> (173.1016, -149.7773) projected
  arc A95 (173.1016, -149.7773) -> (176.1856, -146.1371) centre (0, 0) ccw projected
  line L286 (176.1856, -146.1371) -> (175.0432, -144.1842) projected
  line L287 (175.0432, -144.1842) -> (176.9977, -141.778) projected
  line L288 (176.9977, -141.778) -> (179.1433, -142.4959) projected
  arc A96 (179.1433, -142.4959) -> (182.0742, -138.7314) centre (0, 0) ccw projected
  line L289 (182.0742, -138.7314) -> (180.8521, -136.8274) projected
  line L290 (180.8521, -136.8274) -> (182.7055, -134.3425) projected
  line L291 (182.7055, -134.3425) -> (184.8789, -134.9711) projected
  arc A97 (184.8789, -134.9711) -> (187.6517, -131.0887) centre (0, 0) ccw projected
  line L292 (187.6517, -131.0887) -> (186.352, -129.2368) projected
  line L293 (186.352, -129.2368) -> (188.1011, -126.6774) projected
  line L294 (188.1011, -126.6774) -> (190.2987, -127.2157) projected
  arc A98 (190.2987, -127.2157) -> (192.9086, -123.222) centre (0, 0) ccw projected
  line L295 (192.9086, -123.222) -> (191.5335, -121.4254) projected
  line L296 (191.5335, -121.4254) -> (193.1754, -118.7959) projected
  line L297 (193.1754, -118.7959) -> (195.3933, -119.2429) projected
  arc A99 (195.3933, -119.2429) -> (197.836, -115.1448) centre (0, 0) ccw projected
  line L298 (197.836, -115.1448) -> (196.3878, -113.4066) projected
  line L299 (196.3878, -113.4066) -> (197.9196, -110.7115) projected
  line L300 (197.9196, -110.7115) -> (200.1541, -111.0664) projected
  arc A100 (200.1541, -111.0664) -> (202.4254, -106.8709) centre (0, 0) ccw projected
  line L301 (202.4254, -106.8709) -> (200.9065, -105.194) projected
  line L302 (200.9065, -105.194) -> (202.3257, -102.4379) projected
  line L303 (202.3257, -102.4379) -> (204.5729, -102.7002) projected
  arc A101 (204.5729, -102.7002) -> (206.6689, -98.4143) centre (0, 0) ccw projected
  line L304 (206.6689, -98.4143) -> (205.0821, -96.8017) projected
  line L305 (205.0821, -96.8017) -> (206.3861, -93.9893) projected
  line L306 (206.3861, -93.9893) -> (208.6422, -94.1585) projected
  arc A102 (208.6422, -94.1585) -> (210.5593, -89.7897) centre (0, 0) ccw projected
  line L307 (210.5593, -89.7897) -> (208.9072, -88.244) projected
  line L308 (208.9072, -88.244) -> (210.0939, -85.3801) projected
  line L309 (210.0939, -85.3801) -> (212.3551, -85.4559) projected
  arc A103 (212.3551, -85.4559) -> (214.09, -81.0116) centre (0, 0) ccw projected
  line L310 (214.09, -81.0116) -> (212.3754, -79.5355) projected
  line L311 (212.3754, -79.5355) -> (213.4428, -76.625) projected
  line L312 (213.4428, -76.625) -> (215.7052, -76.6074) projected
  arc A104 (215.7052, -76.6074) -> (217.2549, -72.0952) centre (0, 0) ccw projected
  line L313 (217.2549, -72.0952) -> (215.4808, -70.6911) projected
  line L314 (215.4808, -70.6911) -> (216.427, -67.7391) projected
  line L315 (216.427, -67.7391) -> (218.6867, -67.6279) projected
  arc A105 (218.6867, -67.6279) -> (220.0486, -63.0555) centre (0, 0) ccw projected
  line L316 (220.0486, -63.0555) -> (218.218, -61.726) projected
  line L317 (218.218, -61.726) -> (219.0414, -58.7374) projected
  line L318 (219.0414, -58.7374) -> (221.2946, -58.5329) projected
  arc A106 (221.2946, -58.5329) -> (222.4664, -53.9082) centre (0, 0) ccw projected
  line L319 (222.4664, -53.9082) -> (220.5825, -52.6554) projected
  line L320 (220.5825, -52.6554) -> (221.2816, -49.6353) projected
  line L321 (221.2816, -49.6353) -> (223.5244, -49.3379) projected
  arc A107 (223.5244, -49.3379) -> (224.5042, -44.6687) centre (0, 0) ccw projected
  line L322 (224.5042, -44.6687) -> (222.57, -43.4949) projected
  line L323 (222.57, -43.4949) -> (223.1438, -40.4484) projected
  line L324 (223.1438, -40.4484) -> (225.3724, -40.0586) projected
  arc A108 (225.3724, -40.0586) -> (226.1583, -35.3529) centre (0, 0) ccw projected
  line L325 (226.1583, -35.3529) -> (224.1773, -34.26) projected
  line L326 (224.1773, -34.26) -> (224.6247, -31.1925) projected
  line L327 (224.6247, -31.1925) -> (226.8353, -30.7109) projected
  arc A109 (226.8353, -30.7109) -> (227.4261, -25.9767) centre (0, 0) ccw projected
  line L328 (227.4261, -25.9767) -> (225.4016, -24.9666) projected
  line L329 (225.4016, -24.9666) -> (225.7218, -21.8832) projected
  line L330 (225.7218, -21.8832) -> (227.9106, -21.3107) projected
  arc A110 (227.9106, -21.3107) -> (228.3053, -16.5561) centre (0, 0) ccw projected
  line L331 (228.3053, -16.5561) -> (226.2408, -15.6306) projected
  line L332 (226.2408, -15.6306) -> (226.4333, -12.5366) projected
  line L333 (226.4333, -12.5366) -> (228.5966, -11.8741) projected
  arc A111 (228.5966, -11.8741) -> (228.7944, -7.1073) centre (0, 0) ccw projected
  line L334 (228.7944, -7.1073) -> (226.6935, -6.2678) projected
  line L335 (226.6935, -6.2678) -> (226.758, -3.1685) projected
  line L336 (226.758, -3.1685) -> (228.892, -2.4172) projected
  arc A112 (228.892, -2.4172) -> (228.8927, 2.3537) centre (0, 0) ccw projected
  line L337 (228.8927, 2.3537) -> (226.7588, 3.1056) projected
  line L338 (226.7588, 3.1056) -> (226.6952, 6.205) projected
  line L339 (226.6952, 6.205) -> (228.7964, 7.0438) projected
  arc A113 (228.7964, 7.0438) -> (228.5999, 11.8107) centre (0, 0) ccw projected
  line L340 (228.5999, 11.8107) -> (226.4368, 12.4738) projected
  line L341 (226.4368, 12.4738) -> (226.2451, 15.5678) projected
  line L342 (226.2451, 15.5678) -> (228.3099, 16.4928) projected
  arc A114 (228.3099, 16.4928) -> (227.9165, 21.2475) centre (0, 0) ccw projected
  line L343 (227.9165, 21.2475) -> (225.7279, 21.8206) projected
  line L344 (225.7279, 21.8206) -> (225.4085, 24.9041) projected
  line L345 (225.4085, 24.9041) -> (227.4333, 25.9136) projected
  arc A115 (227.4333, 25.9136) -> (226.8438, 30.648) centre (0, 0) ccw projected
  line L346 (226.8438, 30.648) -> (224.6333, 31.1302) projected
  line L347 (224.6333, 31.1302) -> (224.1868, 34.1978) projected
  line L348 (224.1868, 34.1978) -> (226.1681, 35.2902) projected
  arc A116 (226.1681, 35.2902) -> (225.3835, 39.9961) centre (0, 0) ccw projected
  line L349 (225.3835, 39.9961) -> (223.155, 40.3865) projected
  line L350 (223.155, 40.3865) -> (222.5821, 43.4331) projected
  line L351 (222.5821, 43.4331) -> (224.5165, 44.6064) projected
  arc A117 (224.5165, 44.6064) -> (223.5381, 49.2759) centre (0, 0) ccw projected
  line L352 (223.5381, 49.2759) -> (221.2954, 49.5739) projected
  line L353 (221.2954, 49.5739) -> (220.5971, 52.5942) projected
  line L354 (220.5971, 52.5942) -> (222.4814, 53.8464) projected
  arc A118 (222.4814, 53.8464) -> (221.3108, 58.4715) centre (0, 0) ccw projected
  line L355 (221.3108, 58.4715) -> (219.0577, 58.6766) projected
  line L356 (219.0577, 58.6766) -> (218.2352, 61.6655) projected
  line L357 (218.2352, 61.6655) -> (220.0661, 62.9945) projected
  arc A119 (220.0661, 62.9945) -> (218.7055, 67.5672) centre (0, 0) ccw projected
  line L358 (218.7055, 67.5672) -> (216.4458, 67.679) projected
  line L359 (216.4458, 67.679) -> (215.5004, 70.6313) projected
  line L360 (215.5004, 70.6313) -> (217.2749, 72.0349) projected
  arc A120 (217.2749, 72.0349) -> (215.7264, 76.5475) centre (0, 0) ccw projected
  line L361 (215.7264, 76.5475) -> (213.464, 76.5658) projected
  line L362 (213.464, 76.5658) -> (212.3975, 79.4766) projected
  line L363 (212.3975, 79.4766) -> (214.1125, 80.9522) projected
  arc A121 (214.1125, 80.9522) -> (212.3788, 85.397) centre (0, 0) ccw projected
  line L364 (212.3788, 85.397) -> (210.1176, 85.3218) projected
  line L365 (210.1176, 85.3218) -> (208.9317, 88.186) projected
  line L366 (208.9317, 88.186) -> (210.5842, 89.7313) projected
  arc A122 (210.5842, 89.7313) -> (208.6684, 94.1006) centre (0, 0) ccw projected
  line L367 (208.6684, 94.1006) -> (206.4122, 93.932) projected
  line L368 (206.4122, 93.932) -> (205.1089, 96.7448) projected
  line L369 (205.1089, 96.7448) -> (206.6962, 98.357) projected
  arc A123 (206.6962, 98.357) -> (204.6014, 102.6434) centre (0, 0) ccw projected
  line L370 (204.6014, 102.6434) -> (202.3541, 102.3818) projected
  line L371 (202.3541, 102.3818) -> (200.9357, 105.1382) projected
  line L372 (200.9357, 105.1382) -> (202.455, 106.8147) projected
  arc A124 (202.455, 106.8147) -> (200.1849, 111.0109) centre (0, 0) ccw projected
  line L373 (200.1849, 111.0109) -> (197.9503, 110.6566) projected
  line L374 (197.9503, 110.6566) -> (196.4192, 113.3521) projected
  line L375 (196.4192, 113.3521) -> (197.8679, 115.0899) projected
  arc A125 (197.8679, 115.0899) -> (195.4264, 119.1887) centre (0, 0) ccw projected
  line L376 (195.4264, 119.1887) -> (193.2084, 118.7423) projected
  line L377 (193.2084, 118.7423) -> (191.5672, 121.3723) projected
  line L378 (191.5672, 121.3723) -> (192.9428, 123.1685) projected
  arc A126 (192.9428, 123.1685) -> (190.3339, 127.1629) centre (0, 0) ccw projected
  line L379 (190.3339, 127.1629) -> (188.1363, 126.6252) projected
  line L380 (188.1363, 126.6252) -> (186.3878, 129.1851) projected
  line L381 (186.3878, 129.1851) -> (187.6881, 131.0366) projected
  arc A127 (187.6881, 131.0366) -> (184.9163, 134.9198) centre (0, 0) ccw projected
  line L382 (184.9163, 134.9198) -> (182.7428, 134.2918) projected
  line L383 (182.7428, 134.2918) -> (180.89, 136.7772) projected
  line L384 (180.89, 136.7772) -> (182.1127, 138.6809) projected
  arc A128 (182.1127, 138.6809) -> (179.1828, 142.4462) centre (0, 0) ccw projected
  line L385 (179.1828, 142.4462) -> (177.0371, 141.7289) projected
  line L386 (177.0371, 141.7289) -> (175.0832, 144.1357) projected
  line L387 (175.0832, 144.1357) -> (176.2261, 146.0882) projected
  arc A129 (176.2261, 146.0882) -> (173.1432, 149.7292) centre (0, 0) ccw projected
  line L388 (173.1432, 149.7292) -> (171.0289, 148.9239) projected
  line L389 (171.0289, 148.9239) -> (168.9772, 151.2478) projected
  line L390 (168.9772, 151.2478) -> (170.0385, 153.246) projected
  arc A130 (170.0385, 153.246) -> (166.8077, 156.7565) centre (0, 0) ccw projected
  line L391 (166.8077, 156.7565) -> (164.7285, 155.8644) projected
  line L392 (164.7285, 155.8644) -> (162.5826, 158.1016) projected
  line L393 (162.5826, 158.1016) -> (163.5603, 160.1419) projected
  arc A131 (163.5603, 160.1419) -> (160.1873, 163.5159) centre (0, 0) ccw projected
  line L394 (160.1873, 163.5159) -> (158.1467, 162.5387) projected
  line L395 (158.1467, 162.5387) -> (155.9101, 164.6853) projected
  line L396 (155.9101, 164.6853) -> (156.8028, 166.7642) projected
  arc A132 (156.8028, 166.7642) -> (153.2931, 169.9959) centre (0, 0) ccw projected
  line L397 (153.2931, 169.9959) -> (151.2947, 168.9353) projected
  line L398 (151.2947, 168.9353) -> (148.9713, 170.9876) projected
  line L399 (148.9713, 170.9876) -> (149.7773, 173.1016) projected
  arc A133 (149.7773, 173.1016) -> (146.1371, 176.1856) centre (0, 0) ccw projected
  line L400 (146.1371, 176.1856) -> (144.1842, 175.0432) projected
  line L401 (144.1842, 175.0432) -> (141.778, 176.9977) projected
  line L402 (141.778, 176.9977) -> (142.4959, 179.1433) projected
  arc A134 (142.4959, 179.1433) -> (138.7314, 182.0742) centre (0, 0) ccw projected
  line L403 (138.7314, 182.0742) -> (136.8274, 180.8521) projected
  line L404 (136.8274, 180.8521) -> (134.3425, 182.7055) projected
  line L405 (134.3425, 182.7055) -> (134.9711, 184.8789) projected
  arc A135 (134.9711, 184.8789) -> (131.0887, 187.6517) centre (0, 0) ccw projected
  line L406 (131.0887, 187.6517) -> (129.2368, 186.352) projected
  line L407 (129.2368, 186.352) -> (126.6774, 188.1011) projected
  line L408 (126.6774, 188.1011) -> (127.2157, 190.2987) projected
  arc A136 (127.2157, 190.2987) -> (123.222, 192.9086) centre (0, 0) ccw projected
  line L409 (123.222, 192.9086) -> (121.4254, 191.5335) projected
  line L410 (121.4254, 191.5335) -> (118.7959, 193.1754) projected
  line L411 (118.7959, 193.1754) -> (119.2429, 195.3933) projected
  arc A137 (119.2429, 195.3933) -> (115.1448, 197.836) centre (0, 0) ccw projected
  line L412 (115.1448, 197.836) -> (113.4066, 196.3878) projected
  line L413 (113.4066, 196.3878) -> (110.7115, 197.9196) projected
  line L414 (110.7115, 197.9196) -> (111.0664, 200.1541) projected
  arc A138 (111.0664, 200.1541) -> (106.8709, 202.4254) centre (0, 0) ccw projected
  line L415 (106.8709, 202.4254) -> (105.194, 200.9065) projected
  line L416 (105.194, 200.9065) -> (102.4379, 202.3257) projected
  line L417 (102.4379, 202.3257) -> (102.7002, 204.5729) projected
  arc A139 (102.7002, 204.5729) -> (98.4143, 206.6689) centre (0, 0) ccw projected
  line L418 (98.4143, 206.6689) -> (96.8017, 205.0821) projected
  line L419 (96.8017, 205.0821) -> (93.9893, 206.3861) projected
  line L420 (93.9893, 206.3861) -> (94.1585, 208.6422) projected
  arc A140 (94.1585, 208.6422) -> (89.7897, 210.5593) centre (0, 0) ccw projected
  line L421 (89.7897, 210.5593) -> (88.244, 208.9072) projected
  line L422 (88.244, 208.9072) -> (85.3801, 210.0939) projected
  line L423 (85.3801, 210.0939) -> (85.4559, 212.3551) projected
  arc A141 (85.4559, 212.3551) -> (81.0116, 214.09) centre (0, 0) ccw projected
  line L424 (81.0116, 214.09) -> (79.5355, 212.3754) projected
  line L425 (79.5355, 212.3754) -> (76.625, 213.4428) projected
  line L426 (76.625, 213.4428) -> (76.6074, 215.7052) projected
  arc A142 (76.6074, 215.7052) -> (72.0952, 217.2549) centre (0, 0) ccw projected
  line L427 (72.0952, 217.2549) -> (70.6911, 215.4808) projected
  line L428 (70.6911, 215.4808) -> (67.7391, 216.427) projected
  line L429 (67.7391, 216.427) -> (67.6279, 218.6867) projected
  arc A143 (67.6279, 218.6867) -> (63.0555, 220.0486) centre (0, 0) ccw projected
  line L430 (63.0555, 220.0486) -> (61.726, 218.218) projected
  line L431 (61.726, 218.218) -> (58.7374, 219.0414) projected
  line L432 (58.7374, 219.0414) -> (58.5329, 221.2946) projected
  arc A144 (58.5329, 221.2946) -> (53.9082, 222.4664) centre (0, 0) ccw projected
  line L433 (53.9082, 222.4664) -> (52.6554, 220.5825) projected
  line L434 (52.6554, 220.5825) -> (49.6353, 221.2816) projected
  line L435 (49.6353, 221.2816) -> (49.3379, 223.5244) projected
  arc A145 (49.3379, 223.5244) -> (44.6687, 224.5042) centre (0, 0) ccw projected
  line L436 (44.6687, 224.5042) -> (43.4949, 222.57) projected
  line L437 (43.4949, 222.57) -> (40.4484, 223.1438) projected
  line L438 (40.4484, 223.1438) -> (40.0586, 225.3724) projected
  arc A146 (40.0586, 225.3724) -> (35.3529, 226.1583) centre (0, 0) ccw projected
  line L439 (35.3529, 226.1583) -> (34.26, 224.1773) projected
  line L440 (34.26, 224.1773) -> (31.1925, 224.6247) projected
  line L441 (31.1925, 224.6247) -> (30.7109, 226.8353) projected
  arc A147 (30.7109, 226.8353) -> (25.9767, 227.4261) centre (0, 0) ccw projected
  line L442 (25.9767, 227.4261) -> (24.9666, 225.4016) projected
  line L443 (24.9666, 225.4016) -> (21.8832, 225.7218) projected
  line L444 (21.8832, 225.7218) -> (21.3107, 227.9106) projected
  arc A148 (21.3107, 227.9106) -> (16.5561, 228.3053) centre (0, 0) ccw projected
  line L445 (16.5561, 228.3053) -> (15.6306, 226.2408) projected
  line L446 (15.6306, 226.2408) -> (12.5366, 226.4333) projected
  line L447 (12.5366, 226.4333) -> (11.8741, 228.5966) projected
  arc A149 (11.8741, 228.5966) -> (7.1073, 228.7944) centre (0, 0) ccw projected
  line L448 (7.1073, 228.7944) -> (6.2678, 226.6935) projected
  line L449 (6.2678, 226.6935) -> (3.1685, 226.758) projected
  line L450 (3.1685, 226.758) -> (2.4172, 228.892) projected
  arc A150 (2.4172, 228.892) -> (-11.8107, 228.5999) centre (0, 0) ccw projected
  line L451 (-11.8107, 228.5999) -> (-12.4738, 226.4368) projected
  line L452 (-12.4738, 226.4368) -> (-15.5678, 226.2451) projected
  circle A151 centre (0, 0) radius 236.22
  circle A152 centre (0, 0) radius 223.52
  dimension "d96" = 472.44
  dimension "d97" = 447.04
  constraints: 2 centre point, 2 coincident
  measures "d96" diameter of A151
  measures "d97" diameter of A152
extrude "Extrusion13" add sketch "Sketch17" against normal blind 2.54 contours A151 bodies 2